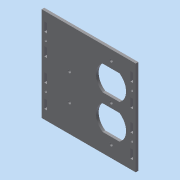
# Autodesk Inventor part: Box Back
Saved by Autodesk Inventor 2013 (Build 170138000, 138)
## iProperties
Created: 2012-12-29
Part Number: Box Back
Material: Generic
Document SubType Name: Modeling
Designer: Administrator
Density: 1 g/cm^3
Author: Administrator
Autodesk Inventor part; units mm, degrees
ref_plane "YZ Plane" through (0, 0, 0) normal (1, 0, 0) x (0, 1, 0)
ref_plane "XZ Plane" through (0, 0, 0) normal (0, 1, 0) x (-1, 0, 0)
ref_plane "XY Plane" through (0, 0, 0) normal (0, 0, 1) x (1, 0, 0)
sketch "Sketch1" plane through (0, 0, 0) normal (0, 0, 1) x (1, 0, 0)
  line L0 (-55.88, 55.88) -> (50.8, 55.88)
  line L1 (50.8, 55.88) -> (50.8, -50.8)
  line L2 (50.8, -50.8) -> (-55.88, -50.8)
  line L3 (-55.88, -50.8) -> (-55.88, 55.88)
  line L4 (13.1719, 37.1163) -> (32.4118, 37.1163)
  line L5 (32.4118, 8.9477) -> (13.1719, 8.9477)
  line L6 (13.1719, -1.7711) -> (32.4118, -1.7711)
  line L7 (32.4118, -29.9397) -> (13.1719, -29.9397)
  circle A0 centre (22.7918, 44.7363) radius 1.778
  circle A1 centre (22.7918, 3.645) radius 1.778
  circle A2 centre (22.7918, -37.5597) radius 1.778
  circle A3 centre (-24.4861, -19.8716) radius 1.778
  circle A4 centre (-24.4861, 10.6084) radius 1.778
  arc A5 (13.1719, 37.1163) -> (13.1719, 8.9477) centre (22.7918, 23.032) ccw
  arc A6 (32.4118, 8.9477) -> (32.4118, 37.1163) centre (22.7918, 23.032) ccw
  arc A7 (13.1719, -1.7711) -> (13.1719, -29.9397) centre (22.7918, -15.8554) ccw
  arc A8 (32.4118, -29.9397) -> (32.4118, -1.7711) centre (22.7918, -15.8554) ccw
  circle A9 centre (-51.38, 27.48) radius 1.525
  circle A10 centre (-51.38, -22.4) radius 1.525
  circle A11 centre (46.3, -22.4) radius 1.525
  circle A12 centre (46.3, 27.48) radius 1.525
  point P0 (0, 0)
  dimension "d0" = 106.68
  dimension "d1" = 106.68
  dimension "d12" = 3.556
  dimension "d13" = 3.556
  dimension "d21" = 3.556
  dimension "d22" = 3.556
  dimension "d24" = 30.48
  dimension "d29" = 28.1686
  dimension "d32" = 3.05
  dimension "d33" = 28.4
  dimension "d34" = 4.5
  dimension "d35" = 3.05
  dimension "d36" = 4.5
  dimension "d37" = 28.4
  dimension "d38" = 3.05
  dimension "d39" = 4.5
  dimension "d40" = 28.4
  dimension "d41" = 3.05
  dimension "d42" = 28.4
  dimension "d43" = 4.5
  constraints: 16 end point, 13 centre point, 8 point on circle, 4 parallel, 3 horizontal, 1 perpendicular
  measures "d0" distance of L1.end L2.end
  measures "d1" distance of L0.end L1.end
  measures "d12" diameter of A1
  measures "d13" diameter of A2
  measures "d21" diameter of A3
  measures "d22" diameter of A4
  measures "d24" distance of A4.centre A3.centre
  measures "d29" distance between parallel lines of L5 L4
  measures "d32" diameter of A9
  measures "d33" distance from line of L0 A9.centre
  measures "d34" distance from line of L3 A9.centre
  measures "d35" diameter of A10
  measures "d36" distance from line of L3 A10.centre
  measures "d37" distance from line of L2 A10.centre
  measures "d38" diameter of A11
  measures "d39" distance from line of L1 A11.centre
  measures "d40" distance from line of L2 A11.centre
  measures "d41" diameter of A12
  measures "d42" distance from line of L0 A12.centre
  measures "d43" distance from line of L1 A12.centre
extrude "Extrusion2" add sketch "Sketch1" along normal blind 3
sketch "Sketch2" plane through (0, 0, 3) normal (0, 0, 1) x (1, 0, 0)
  circle A0 centre (46.3, 27.48) radius 1.525 projected
  circle A1 centre (46.3, -22.4) radius 1.525 projected
  circle A2 centre (-51.38, -22.4) radius 1.525 projected
  circle A3 centre (-51.38, 27.48) radius 1.525 projected
  line L0 (-49.7999, 35.305) -> (-52.8999, 35.305)
  line L1 (-52.8999, 35.305) -> (-52.8999, 45.405)
  line L2 (-52.8999, 45.405) -> (-49.7999, 45.405)
  line L3 (-49.7999, 45.405) -> (-49.7999, 35.305)
  line L4 (-49.7999, 21.18) -> (-52.8999, 21.18)
  line L5 (-52.8999, 21.18) -> (-52.8999, 11.08)
  line L6 (-52.8999, 11.08) -> (-49.7999, 11.08)
  line L7 (-49.7999, 11.08) -> (-49.7999, 21.18)
  line L8 (-49.7999, -4.475) -> (-52.8999, -4.475)
  line L9 (-52.8999, -4.475) -> (-52.8999, -14.575)
  line L10 (-52.8999, -14.575) -> (-49.7999, -14.575)
  line L11 (-49.7999, -14.575) -> (-49.7999, -4.475)
  line L12 (-49.7999, -30.225) -> (-52.8999, -30.225)
  line L13 (-52.8999, -30.225) -> (-52.8999, -40.325)
  line L14 (-52.8999, -40.325) -> (-49.7999, -40.325)
  line L15 (-49.7999, -40.325) -> (-49.7999, -30.225)
  line L16 (47.825, -30.225) -> (44.725, -30.225)
  line L17 (44.725, -30.225) -> (44.725, -40.325)
  line L18 (44.725, -40.325) -> (47.825, -40.325)
  line L19 (47.825, -40.325) -> (47.825, -30.225)
  line L20 (47.825, -14.575) -> (44.725, -14.575)
  line L21 (44.725, -14.575) -> (44.725, -4.475)
  line L22 (44.725, -4.475) -> (47.825, -4.475)
  line L23 (47.825, -4.475) -> (47.825, -14.575)
  line L24 (47.85, 35.305) -> (44.75, 35.305)
  line L25 (44.75, 35.305) -> (44.75, 45.405)
  line L26 (44.75, 45.405) -> (47.85, 45.405)
  line L27 (47.85, 45.405) -> (47.85, 35.305)
  line L28 (47.8453, 19.655) -> (44.7453, 19.655)
  line L29 (44.7453, 19.655) -> (44.7453, 9.555)
  line L30 (44.7453, 9.555) -> (47.8453, 9.555)
  line L31 (47.8453, 9.555) -> (47.8453, 19.655)
  point P0 (0, 0)
  dimension "d46" = 3.1
  dimension "d47" = 10.1
  dimension "d48" = 3.1
  dimension "d49" = 10.1
  dimension "d50" = 6.3
  dimension "d51" = 6.3
  dimension "d52" = 3.1
  dimension "d53" = 10.1
  dimension "d54" = 3.1
  dimension "d55" = 10.1
  dimension "d58" = 6.3
  dimension "d60" = 6.3
  dimension "d61" = 3.1
  dimension "d62" = 10.1
  dimension "d63" = 3.1
  dimension "d64" = 10.1
  dimension "d65" = 6.3
  dimension "d66" = 6.3
  dimension "d67" = 3.1
  dimension "d68" = 10.1
  dimension "d69" = 3.1
  dimension "d70" = 10.1
  dimension "d71" = 6.3
  dimension "d72" = 6.3
  constraints: 64 end point, 16 parallel, 8 horizontal, 8 perpendicular
  measures "d46" distance of L1.end L2.end
  measures "d47" distance of L0.end L1.end
  measures "d48" distance of L6.end L5.end
  measures "d49" distance of L5.end L4.end
  measures "d50" distance edge to line of A3 L0
  measures "d51" distance from line of L4 A3.centre
  measures "d52" distance of L10.end L9.end
  measures "d53" distance of L9.end L8.end
  measures "d54" distance of L14.end L13.end
  measures "d55" distance of L13.end L12.end
  measures "d58" distance edge to line of A2 L12
  measures "d60" distance edge to line of A2 L10
  measures "d61" distance of L18.end L17.end
  measures "d62" distance of L17.end L16.end
  measures "d63" distance of L21.end L22.end
  measures "d64" distance of L20.end L21.end
  measures "d65" distance edge to line of A1 L20
  measures "d66" distance edge to line of A1 L16
  measures "d67" distance of L25.end L26.end
  measures "d68" distance of L24.end L25.end
  measures "d69" distance of L30.end L29.end
  measures "d70" distance of L29.end L28.end
  measures "d71" distance edge to line of A0 L28
  measures "d72" distance edge to line of A0 L24
extrude "Extrusion3" cut sketch "Sketch2" against normal through all contours L0 L1 L2 L3 | L7 L6 L5 L4 | L11 L10 L9 L8 | L15 L14 L13 L12 | L19 L18 L17 L16 | L20 L21 L22 L23 | L24 L25 L26 L27 | L31 L30 L29 L28
body "Solid2"
